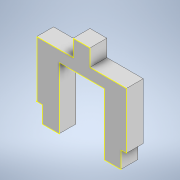
# Autodesk Inventor part: motorbase_1
Saved by Autodesk Inventor 2022 (Build 260153000, 153)
## iProperties
Created: 2023-04-18
Part Number: motorbase_1
Material: 一般
Document SubType Name: Modeling
Designer: Johnny Jou
Density: 1 g/cm^3
Appearance: 預設
Author: Johnny Jou
Autodesk Inventor part; units mm, degrees
ref_plane "YZ Plane" through (0, 0, 0) normal (1, 0, 0) x (0, 1, 0)
ref_plane "XZ Plane" through (0, 0, 0) normal (0, 1, 0) x (-1, 0, 0)
ref_plane "XY Plane" through (0, 0, 0) normal (0, 0, 1) x (1, 0, 0)
sketch "草圖1" plane through (0, 0, 0) normal (0, 0, 1) x (1, 0, 0)
  line L0 (0, 0) -> (16, 0)
  line L1 (16, 0) -> (16, 10)
  line L2 (16, 10) -> (0, 10)
  line L3 (0, 10) -> (0, 0)
  line L4 (4, 0) -> (12, 0)
  line L5 (12, 0) -> (12, 8)
  line L6 (12, 8) -> (4, 8)
  line L7 (4, 8) -> (4, 0)
  line L8 (0, 10) -> (16, 0) construction
  line L9 (16, 10) -> (0, 0) construction
  circle A0 centre (8, 5) radius 1.5 construction
  line L10 (6.5, 10) -> (9.5, 10) construction
  line L11 (9.5, 10) -> (9.5, 13)
  line L12 (9.5, 13) -> (6.5, 13)
  line L13 (6.5, 13) -> (6.5, 10)
  line L14 (4, 0) -> (1, 0)
  line L15 (1, 0) -> (1, -3)
  line L16 (1, -3) -> (4, -3)
  line L17 (4, -3) -> (4, 0)
  line L18 (12, 0) -> (15, 0)
  line L19 (15, 0) -> (15, -3)
  line L20 (15, -3) -> (12, -3)
  line L21 (12, -3) -> (12, 0)
  point P0 (8, 13)
  point P1 (8, 5)
  point P2 (1, 0)
  dimension "d0" = 8
  dimension "d1" = 3
  dimension "d2" = 2
  dimension "d3" = 16
  dimension "d4" = 4
  dimension "d5" = 10
  dimension "d6" = 3
  dimension "d7" = 3
  dimension "d8" = 3
  dimension "d9" = 3
  dimension "d10" = 3
  constraints: 44 end point, 10 parallel, 5 horizontal, 5 perpendicular, 3 midpoint, 3 point on line, 1 centre point, 1 vertical alignment
  measures "d0" distance between parallel lines of L5 L7
  measures "d1" diameter of A0
  measures "d2" distance between parallel lines of L2 L6
  measures "d3" distance between parallel lines of L1 L3
  measures "d4" distance between parallel lines of L1 L5
  measures "d5" distance between parallel lines of L0 L2
  measures "d6" distance of L12.end L10.start
  measures "d7" distance of L11.end L12.end
  measures "d8" distance of L15.end L16.end
  measures "d9" distance of L19.end L20.end
  measures "d10" distance of L18.end L19.end
extrude "擠出1" add sketch "草圖1" along normal blind 3 contours L3 L2 L1 L0 L5 L6 L7 | L0 L17 L16 L15 | L13 L12 L11 L2 | L0 L19 L20 L21
sketch "草圖2" plane through (0, 0, 3) normal (0, 0, 1) x (1, 0, 0)
  line L0 (15, -3) -> (15, 0) projected
  line L1 (15, 0) -> (16, 0) projected
  line L2 (16, 0) -> (16, 10) projected
  line L3 (16, 10) -> (9.5, 10) projected
  line L4 (9.5, 10) -> (9.5, 13) projected
  line L5 (9.5, 13) -> (6.5, 13) projected
  line L6 (6.5, 13) -> (6.5, 10) projected
  line L7 (6.5, 10) -> (0, 10) projected
  line L8 (0, 10) -> (0, 0) projected
  line L9 (0, 0) -> (1, 0) projected
  line L10 (1, 0) -> (1, -3) projected
  line L11 (1, -3) -> (4, -3) projected
  line L12 (4, -3) -> (4, 8) projected
  line L13 (4, 8) -> (12, 8) projected
  line L14 (12, 8) -> (12, -3) projected
  line L15 (12, -3) -> (15, -3) projected
